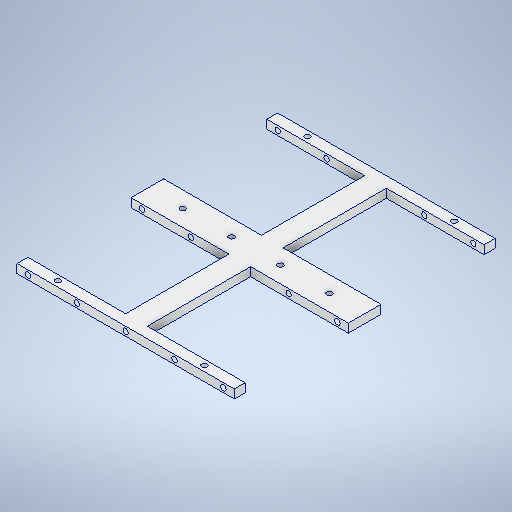
# Autodesk Inventor part: 02
Saved by Autodesk Inventor 2025.1 (Build 291241000, 241)
## iProperties
Created: 2024-09-17
Part Number: 02
Material: Aluminum 6061
Document SubType Name: Modeling
Designer: ffogue
Density: 2.7 g/cm^3
Appearance: Aluminum - Flat
Author: ffogue
Autodesk Inventor part; units mm, degrees
ref_plane "YZ Plane" through (0, 0, 0) normal (1, 0, 0) x (0, 1, 0)
ref_plane "XY Plane" through (0, 0, 0) normal (0, 0, 1) x (1, 0, 0)
sketch "Sketch1" plane through (0, 0, 0) normal (0, 0, 1) x (1, 0, 0)
  line L0 (-10, 135) -> (-10, 230)
  line L1 (-10, 230) -> (-100, 230)
  line L2 (-100, 230) -> (-100, 240)
  line L3 (-100, 240) -> (100, 240)
  line L4 (100, 240) -> (100, 230)
  line L5 (100, 230) -> (10, 230)
  line L6 (10, 230) -> (10, 135)
  line L7 (10, 135) -> (100, 135)
  line L8 (100, 135) -> (100, 105)
  line L9 (100, 105) -> (10, 105)
  line L10 (10, 105) -> (10, 10)
  line L11 (10, 10) -> (100, 10)
  line L12 (100, 10) -> (100, 0)
  line L13 (100, 0) -> (-100, 0)
  line L14 (-100, 0) -> (-100, 10)
  line L15 (-100, 10) -> (-10, 10)
  line L16 (-10, 10) -> (-10, 105)
  line L17 (-10, 105) -> (-100, 105)
  line L18 (-100, 105) -> (-100, 135)
  line L19 (-100, 135) -> (-10, 135)
  line L20 (0, 0) -> (0, 240) construction
  dimension "d0" = 10
  dimension "d1" = 200
  dimension "d2" = 20
  dimension "d3" = 30
  dimension "d4" = 10
  dimension "d5" = 95
  dimension "d6" = 95
  constraints: 42 end point, 17 point on line, 11 perpendicular, 2 midpoint, 2 vertical, 1 coincident, 1 parallel, 1 other
  measures "d0" distance of L13.end L14.end
  measures "d1" distance of L12.end L13.end
  measures "d2" distance between parallel lines of L6 L0
  measures "d3" distance of L17.end L18.end
  measures "d4" distance of L1.end L2.end
  measures "d5" distance between parallel lines of L19 L1
  measures "d6" distance between parallel lines of L15 L17
extrude "Extrusion1" add sketch "Sketch1" against normal blind 8
sketch "Sketch2" plane through (0, 0, 0) normal (0, 0, 1) x (1, 0, 0)
  line L0 (-10, 135) -> (-100, 135) projected
  line L1 (-100, 0) -> (100, 0) projected
  line L2 (-100, 240) -> (-100, 230) projected
  line L3 (-100, 10) -> (-100, 0) projected
  point P0 (0, 0)
  point P1 (-67.5, 120)
  point P2 (-22.5, 120)
  point P3 (22.5, 120)
  point P4 (67.5, 120)
  point P5 (0, 0)
  point P6 (-67.5, 235)
  point P7 (67.5, 235)
  point P8 (67.5, 5)
  point P9 (-67.5, 5)
  point P10 (-100, 235)
  point P11 (-100, 5)
  point P12 (0, 0)
  dimension "d9" = 15
  dimension "d10" = 67.5
  dimension "d11" = 45
  dimension "d12" = 45
  dimension "d13" = 45
  dimension "d14" = 67.5
  dimension "d15" = 135
  constraints: 7 horizontal alignment, 4 midpoint, 2 vertical alignment
  measures "d9" distance from line of L0 point (-67.5, 120)
  measures "d10" horizontal distance of point (0, 0) point (-67.5, 120)
  measures "d11" distance of point (-67.5, 120) point (-22.5, 120)
  measures "d12" distance of point (22.5, 120) point (-22.5, 120)
  measures "d13" distance of point (67.5, 120) point (22.5, 120)
  measures "d14" horizontal distance of point (0, 0) point (-67.5, 235)
  measures "d15" distance of point (67.5, 235) point (-67.5, 235)
hole "Hole1" at (-67.5, 120, 0) at (-22.5, 120, 0) at (22.5, 120, 0) at (67.5, 120, 0) at (-67.5, 235, 0) at (67.5, 235, 0) at (67.5, 5, 0) at (-67.5, 5, 0) direction (0, 0, -1) diameter 5 depth 8
sketch "Sketch3" plane through (-100, 0, 0) normal (0, -1, 0) x (1, 0, 0)
  line L0 (0, 0) -> (200, 0) projected
  line L1 (200, -8) -> (0, -8) projected
  point P0 (100, 0)
  point P1 (10, -4)
  point P2 (55, -4)
  point P3 (145, -4)
  point P4 (190, -4)
  point P5 (100, 0)
  point P6 (100, -4)
  point P7 (100, 0)
  dimension "d23" = 4
  dimension "d24" = 45
  dimension "d25" = 90
  dimension "d26" = 90
  dimension "d27" = 45
  constraints: 5 horizontal alignment, 2 midpoint, 1 vertical alignment
  measures "d23" distance from line of L1 point (10, -4)
  measures "d24" distance of point (55, -4) point (10, -4)
  measures "d25" distance of point (10, -4) point (100, -4)
  measures "d26" distance of point (190, -4) point (100, -4)
  measures "d27" distance of point (100, -4) point (145, -4)
hole "Hole2" at (-90, 0, -4) at (-45, 0, -4) at (45, 0, -4) at (90, 0, -4) at (0, 0, -4) direction (0, 1, 0) diameter 5 depth 10
ref_plane "Work Plane1" through (0, 120, 0) normal (0, 1, 0) x (-1, 0, 0)
mirror "Mirror1" about plane through (0, 120, 0) normal (0, 1, 0) of "Hole2"
sketch "Sketch4" plane through (-100, 105, 0) normal (0, -1, 0) x (1, 0, 0)
  circle A0 centre (100, -4) radius 2.5 projected
  line L0 (0, -8) -> (90, -8) projected
  point P0 (100, 0)
  point P1 (10, -4)
  point P2 (55, -4)
  point P3 (145, -4)
  point P4 (190, -4)
  dimension "d36" = 4
  dimension "d37" = 180
  dimension "d38" = 90
  dimension "d39" = 45
  dimension "d48" = 45
  constraints: 3 horizontal alignment
  measures "d36" distance from line of L0 point (10, -4)
  measures "d37" distance of point (190, -4) point (10, -4)
  measures "d38" distance of A0.centre point (10, -4)
  measures "d39" distance of point (55, -4) point (10, -4)
  measures "d48" distance of point (145, -4) A0.centre
hole "Hole3" at (-90, 105, -4) at (-45, 105, -4) at (45, 105, -4) at (90, 105, -4) direction (0, 1, 0) diameter 5 depth 30
equation "\"d6\" = d5"
equation "\"d12\" = d11"
equation "\"d13\" = d11"
equation "\"d14\" = d10"
equation "\"d26\" = d25"
equation "\"d27\" = d24"
equation "\"d38\" = 0.5 * d37"
equation "\"d39\" = 0.5 * d38"
body "Solid1"
